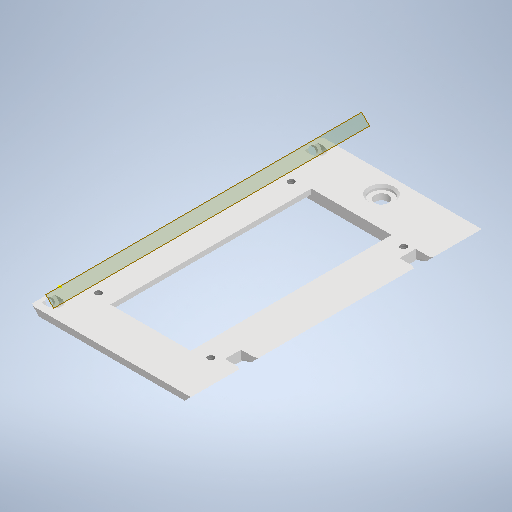
# Autodesk Inventor part: menuDisplay
Saved by Autodesk Inventor 2025 (Build 290162000, 162)
## iProperties
Created: 2024-04-01
Part Number: menuDisplay
Material: Generic
Document SubType Name: Modeling
Designer: 48791
Density: 1 g/cm^3
Appearance: Default
Author: 48791
Autodesk Inventor part; units mm, degrees
ref_plane "YZ Plane" through (0, 0, 0) normal (1, 0, 0) x (0, 1, 0)
ref_plane "XZ Plane" through (0, 0, 0) normal (0, 1, 0) x (-1, 0, 0)
ref_plane "XY Plane" through (0, 0, 0) normal (0, 0, 1) x (1, 0, 0)
sketch "Sketch1" plane through (0, 0, 0) normal (0, 1, 0) x (-1, 0, 0)
  line L0 (0, 0) -> (-80, 0)
  line L1 (-80, 0) -> (-80, -130)
  line L2 (-80, -130) -> (0, -130)
  line L3 (0, -130) -> (0, 0)
  line L4 (-10, -5) -> (-70, -5)
  line L5 (-70, -5) -> (-70, -105)
  line L6 (-70, -105) -> (-10, -105)
  line L7 (-10, -105) -> (-10, -5)
  line L8 (-20, -5) -> (-60, -5)
  line L9 (-60, -5) -> (-60, -105)
  line L10 (-60, -105) -> (-20, -105)
  line L11 (-20, -105) -> (-20, -5)
  circle A0 centre (-40, -120) radius 3.5
  circle A1 centre (-40, -120) radius 5.5
  point P0 (-40, -5)
  point P1 (-40, -105)
  dimension "d0" = 80
  dimension "d1" = 130
  dimension "d2" = 60
  dimension "d3" = 100
  dimension "d4" = 10
  dimension "d5" = 5
  dimension "d6" = 40
  dimension "d7" = 100
  dimension "d8" = 0
  dimension "d9" = 10
  dimension "d10" = 7
  dimension "d11" = 40
  dimension "d12" = 15
  dimension "d66" = 11
  constraints: 24 end point, 6 parallel, 3 horizontal, 3 perpendicular, 2 centre point, 2 midpoint, 1 coincident
  measures "d0" distance of L2.end L1.end
  measures "d1" distance of L1.end L0.end
  measures "d2" distance of L6.end L5.end
  measures "d3" distance of L5.end L4.end
  measures "d4" distance between parallel lines of L7 L3
  measures "d5" distance between parallel lines of L0 L4
  measures "d6" distance of L10.end L9.end
  measures "d7" distance of L9.end L8.end
  measures "d8" distance from line of point (-40, -5) L8
  measures "d9" distance between parallel lines of L7 L11
  measures "d10" diameter of A0
  measures "d11" distance from line of L3 A0.centre
  measures "d12" distance of point (-40, -105) A0.centre
  measures "d66" diameter of A1
extrude "Extrusion1" add sketch "Sketch1" along normal blind 5 contours L3 L2 L1 L0 | A1
sketch "Sketch2" plane through (10, 0, -5) normal (1, 0, 0) x (0, 0, -1)
  line L0 (0, 5) -> (100, 5) projected
  line L1 (100, 0) -> (100, 5) projected
  line L2 (0, 5) -> (100, 5)
  line L3 (100, 5) -> (100, 2.5)
  line L4 (100, 2.5) -> (0, 2.5)
  line L5 (0, 2.5) -> (0, 5)
  point P0 (-5, 0)
  constraints: 8 end point, 2 parallel, 1 horizontal, 1 midpoint, 1 perpendicular
extrude "Extrusion2" add sketch "Sketch2" along normal blind 10
sketch "Sketch3" plane through (70, 0, -105) normal (-1, 0, 0) x (0, 0, 1)
  line L0 (0, 5) -> (100, 5) projected
  line L1 (100, 0) -> (100, 5) projected
  line L2 (0, 5) -> (100, 5)
  line L3 (100, 5) -> (100, 2.5)
  line L4 (100, 2.5) -> (0, 2.5)
  line L5 (0, 2.5) -> (0, 5)
  point P0 (105, 0)
  dimension "d17" = 100
  constraints: 8 end point, 2 parallel, 1 horizontal, 1 midpoint, 1 perpendicular
  measures "d17" distance of L3.end L4.end
extrude "Extrusion3" add sketch "Sketch3" along normal blind 10
sketch "Sketch4" plane through (0, 0, 0) normal (0, 0, 1) x (1, 0, 0)
  point P0 (0, 0)
sketch "Sketch5" plane through (0, 0, 0) normal (0, 0, 1) x (1, 0, 0)
  line L0 (0, 5) -> (80, 5) projected
  line L1 (0, 0) -> (80, 0)
  line L2 (80, 0) -> (80, 5)
  line L3 (80, 5) -> (0, 5)
  line L4 (0, 5) -> (0, 0)
  constraints: 8 end point, 2 parallel, 1 horizontal, 1 perpendicular
extrude "Extrusion4" add sketch "Sketch5" along normal blind 15
sketch "Sketch6" plane through (80, 0, -130) normal (0, 0, -1) x (-1, 0, 0)
  line L0 (0, 5) -> (80, 5) projected
  line L1 (80, 5) -> (80, 0) projected
  line L2 (80, 5) -> (80, 0)
  line L3 (0, 0) -> (0, 5) projected
  line L4 (0, 5) -> (0, 0)
  line L5 (0, 0) -> (5, 0)
  line L6 (5, 0) -> (0, 5)
  dimension "d22" = 5
  constraints: 8 end point, 1 collinear, 1 perpendicular, 1 vertical
  measures "d22" distance of L3.start L5.end
extrude "Extrusion5" cut sketch "Sketch6" against normal blind 210
sketch "Sketch7" plane through (0, 5, 0) normal (0, 1, 0) x (1, 0, 0)
  point P0 (0, 0)
sketch "Sketch8" plane through (0, 0, -130) normal (0, 0, -1) x (-1, 0, 0)
  line L0 (0, 5) -> (0, 0)
  line L1 (0, 0) -> (-5, 0)
  line L2 (-5, 0) -> (0, 5)
  dimension "d25" = 5
  constraints: 6 end point, 1 perpendicular, 1 vertical
  measures "d25" distance of L0.end L1.end
extrude "Extrusion6" cut sketch "Sketch8" against normal blind 210
sketch "Sketch9" plane through (0, 5, 0) normal (0, 1, 0) x (1, 0, 0)
  line L0 (80, 130) -> (80, -15) projected
  line L1 (80, 10) -> (72, 10)
  line L2 (72, 10) -> (72, 16)
  line L3 (72, 16) -> (80, 16)
  line L4 (80, 16) -> (80, 10)
  line L5 (80, 99) -> (72, 99)
  line L6 (72, 99) -> (72, 105)
  line L7 (72, 105) -> (80, 105)
  line L8 (80, 105) -> (80, 99)
  line L9 (5, -15) -> (75, -15) projected
  line L10 (80, 130) -> (0, 130) projected
  point P0 (0, 0)
  point P1 (76, 105)
  dimension "d28" = 8
  dimension "d29" = 6
  dimension "d30" = 8
  dimension "d31" = 6
  dimension "d32" = 25
  dimension "d33" = 25
  constraints: 16 end point, 4 parallel, 2 horizontal, 2 perpendicular, 2 point on line, 1 midpoint
  measures "d28" distance of L2.end L3.end
  measures "d29" distance of L1.end L2.end
  measures "d30" distance of L6.end L7.end
  measures "d31" distance of L5.end L6.end
  measures "d32" distance between parallel lines of L9 L1
  measures "d33" distance from line of L10 point (76, 105)
extrude "Extrusion7" cut sketch "Sketch9" against normal blind 210
sketch "Sketch10" plane through (0, 5, 0) normal (0, 1, 0) x (1, 0, 0)
  point P0 (0, 0)
sketch "Sketch11" plane through (0, 5, 0) normal (0, 1, 0) x (1, 0, 0)
  line L0 (72, 10) -> (72, 16) projected
  line L1 (80, 99) -> (80, 16) projected
  line L2 (72, 16) -> (80, 16)
  line L3 (80, 16) -> (80, 18)
  line L4 (80, 18) -> (72, 18)
  line L5 (72, 18) -> (72, 16)
  line L6 (72, 99) -> (80, 99)
  line L7 (80, 99) -> (80, 97)
  line L8 (80, 97) -> (72, 97)
  line L9 (72, 97) -> (72, 99)
  point P0 (0, 0)
  point P1 (80, 16)
  dimension "d36" = 2
  dimension "d37" = 8
  dimension "d38" = 2
  constraints: 16 end point, 4 parallel, 2 horizontal, 2 perpendicular, 2 point on line
  measures "d36" distance of L3.end L2.end
  measures "d37" distance of L7.end L8.end
  measures "d38" distance of L6.end L7.end
extrude "Extrusion8" cut sketch "Sketch11" against normal blind 20
sketch "Sketch12" plane through (0, 0, 0) normal (0, -1, 0) x (1, 0, 0)
  point P0 (0, 0)
sketch "Sketch13" plane through (70, 2.5, -105) normal (0, -1, 0) x (1, 0, 0)
  circle A0 centre (-2, 98) radius 2
  circle A1 centre (-2, 2) radius 2
  circle A2 centre (-58, 98) radius 2
  circle A3 centre (-58, 2) radius 2
  line L0 (0, 100) -> (0, 0) projected
  line L1 (-10, 100) -> (0, 100) projected
  line L2 (0, 0) -> (-10, 0) projected
  line L3 (-60, 0) -> (-60, 100) projected
  line L4 (-50, 0) -> (-60, 0) projected
  line L5 (-60, 100) -> (-50, 100) projected
  point P0 (-70, 105)
  point P1 (-55, 100)
  dimension "d41" = 4
  dimension "d42" = 4
  dimension "d43" = 4
  dimension "d44" = 4
  dimension "d45" = 2
  dimension "d46" = 2
  dimension "d47" = 0
  dimension "d48" = 2
  dimension "d49" = 2
  dimension "d50" = 2
  dimension "d51" = 2
  dimension "d52" = 2
  constraints: 4 centre point, 1 midpoint
  measures "d41" diameter of A0
  measures "d42" diameter of A1
  measures "d43" diameter of A2
  measures "d44" diameter of A3
  measures "d45" distance from line of L0 A0.centre
  measures "d46" distance from line of L1 A0.centre
  measures "d47" distance edge to line of A1 L0
  measures "d48" distance from line of L2 A1.centre
  measures "d49" distance from line of L3 A3.centre
  measures "d50" distance from line of L4 A3.centre
  measures "d51" vertical distance of point (-55, 100) A2.centre
  measures "d52" distance from line of A2.centre L3
hole "Hole1" at (68, 2.5, -7) at (68, 2.5, -103) at (12, 2.5, -7) at (12, 2.5, -103) direction (0, 1, 0) diameter 3.242 depth 11.8 countersink diameter 4 countersink angle 90 thread size "M4x0.7" class "6H" standard "ANSI Metric M Profile"
chamfer "Chamfer1" distance 2 angle 45 6 edges at (40, 0, 15) (5, 0, -57.5) (40, 0, -130) (75, 0, -57.5) (75, 0, 2.5) (75, 0, -117.5)
chamfer "Chamfer2" distance 1 angle 45 8 edges at (74.7071, 0.7071, -10) (78.2071, 3.2071, -10) (78.2071, 3.2071, -18) (74.7071, 0.7071, -18) (78.2071, 3.2071, -105) (74.7071, 0.7071, -105) (74.7071, 0.7071, -97) (78.2071, 3.2071, -97)
sketch "Sketch14" plane through (0, 5, 0) normal (0, 1, 0) x (1, 0, 0)
  line L0 (78.5858, 97) -> (80, 96) projected
  line L1 (80, 96) -> (80, 19) projected
  line L2 (80, 19) -> (78.5858, 18) projected
  line L3 (78.5858, 18) -> (72, 18) projected
  line L4 (72, 18) -> (72, 10) projected
  line L5 (72, 10) -> (78.5858, 10) projected
  line L6 (78.5858, 10) -> (80, 9) projected
  line L7 (80, 9) -> (80, -15) projected
  line L8 (80, -15) -> (0, -15) projected
  line L9 (0, -15) -> (0, 130) projected
  line L10 (0, 130) -> (80, 130) projected
  line L11 (80, 130) -> (80, 106) projected
  line L12 (80, 106) -> (78.5858, 105) projected
  line L13 (78.5858, 105) -> (72, 105) projected
  line L14 (72, 105) -> (72, 97) projected
  line L15 (72, 97) -> (78.5858, 97) projected
  circle A0 centre (40, 120) radius 3.5 projected
  line L16 (60, 5) -> (60, 105) projected
  line L17 (60, 105) -> (20, 105) projected
  line L18 (20, 105) -> (20, 5) projected
  line L19 (20, 5) -> (60, 5) projected
  circle A1 centre (68, 7) radius 1.621 projected
  circle A2 centre (68, 103) radius 1.621 projected
  circle A3 centre (12, 7) radius 1.621 projected
  circle A4 centre (12, 103) radius 1.621 projected
  circle A5 centre (40, 120) radius 5.5
  point P0 (0, 0)
  dimension "d67" = 11
  constraints: 1 centre point, 1 coincident
  measures "d67" diameter of A5
extrude "Extrusion9" cut sketch "Sketch14" against normal blind 2 contours A5
chamfer "Chamfer3" distance 1 angle 45 1 edges at (34.5, 5, -120)
chamfer "Chamfer4" distance 1 angle 45 2 edges at (1.5, 3.5, -130) (1.5, 3.5, 15)
sketch "Sketch15" plane through (0, 5, 14) normal (-0.7071068, -0.7071068, 0) x (-0.7071068, 0.7071068, 0)
  circle A0 centre (-2.8585, 137) radius 1.6 projected
  circle A1 centre (-2.8585, 6) radius 1.6 projected
  circle A2 centre (-2.8585, 137) radius 2
  circle A3 centre (-2.8585, 6) radius 2
  point P0 (-3.5355, 14)
  dimension "d76" = 4
  dimension "d77" = 4
  constraints: 2 centre point, 2 coincident
  measures "d76" diameter of A2
  measures "d77" diameter of A3
extrude "Extrusion10" cut sketch "Sketch15" against normal blind 25.8125 contours A0 | A1 | A2 | A3
ref_plane "Work Plane1" through (14.1421, 19.1421, 14) normal (-0.7071068, -0.7071068, 0) x (-0.7071068, 0.7071068, 0)
sketch "Sketch16" plane through (0, 5, 0) normal (0, 1, 0) x (1, 0, 0)
  point P0 (0, 0)
sketch "Sketch17" plane through (14.1421, 19.1421, 14) normal (-0.7071068, -0.7071068, 0) x (-0.7071068, 0.7071068, 0)
  circle A0 centre (-2.8585, 137) radius 2 projected
  circle A1 centre (-2.8585, 6) radius 2 projected
  line L0 (-1, -1) -> (0, 0) projected
  line L1 (-56.5685, -1) -> (-1, -1) projected
  line L2 (-56.5685, 23) -> (-56.5685, -1) projected
  line L3 (-55.5685, 24) -> (-56.5685, 23) projected
  line L4 (-55.5685, 24) -> (-50.9117, 24) projected
  line L5 (-50.9117, 24) -> (-50.9117, 32) projected
  line L6 (-50.9117, 32) -> (-55.5685, 32) projected
  line L7 (-56.5685, 33) -> (-55.5685, 32) projected
  line L8 (-56.5685, 110) -> (-56.5685, 33) projected
  line L9 (-55.5685, 111) -> (-56.5685, 110) projected
  line L10 (-55.5685, 111) -> (-50.9117, 111) projected
  line L11 (-50.9117, 111) -> (-50.9117, 119) projected
  line L12 (-50.9117, 119) -> (-55.5685, 119) projected
  line L13 (-56.5685, 120) -> (-55.5685, 119) projected
  line L14 (-56.5685, 144) -> (-56.5685, 120) projected
  line L15 (-56.5685, 144) -> (-1, 144) projected
  line L16 (0, 143) -> (-1, 144) projected
  line L17 (0, 143) -> (0, 0) projected
  ellipse E0 centre (-8.4853, 117) end of major axis (-8.4853, 115.379) minor radius 1.1462 projected
  ellipse E1 centre (-8.4853, 21) end of major axis (-8.4853, 19.379) minor radius 1.1462 projected
  ellipse E2 centre (-48.0833, 117) end of major axis (-48.0833, 115.379) minor radius 1.1462 projected
  ellipse E3 centre (-48.0833, 21) end of major axis (-48.0833, 19.379) minor radius 1.1462 projected
  line L18 (-42.4264, 19) -> (-42.4264, 119) projected
  line L19 (-42.4264, 19) -> (-14.1421, 19) projected
  line L20 (-14.1421, 119) -> (-14.1421, 19) projected
  line L21 (-14.1421, 119) -> (-42.4264, 119) projected
  ellipse E4 centre (-28.2843, 134) end of major axis (-28.2843, 127.5) minor radius 4.5962 projected
  circle A2 centre (-2.8585, 6) radius 3.5
  circle A3 centre (-2.8585, 137) radius 3.5
  point P0 (-3.5355, 14)
  dimension "d81" = 7
  dimension "d82" = 7
  constraints: 2 centre point, 2 coincident, 5 other
  measures "d81" diameter of A2
  measures "d82" diameter of A3
extrude "Extrusion11" cut sketch "Sketch17" along normal blind 18.6375 contours A0 | A1 | A2 L17 | L17 A2 | A3 L17 | L17 A3
body "Solid1"
